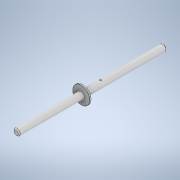
# Autodesk Inventor part: Handle
Saved by Autodesk Inventor 2022 (Build 260153000, 153)
## iProperties
Created: 2022-04-12
Part Number: Handle
Material: Generic
Document SubType Name: Modeling
Designer: Patrick
Density: 1 g/cm^3
Appearance: Default
Author: Patrick
Autodesk Inventor part; units mm, degrees
ref_plane "YZ Plane" through (0, 0, 0) normal (1, 0, 0) x (0, 1, 0)
ref_plane "XZ Plane" through (0, 0, 0) normal (0, 1, 0) x (-1, 0, 0)
ref_plane "XY Plane" through (0, 0, 0) normal (0, 0, 1) x (1, 0, 0)
sketch "Sketch1" plane through (0, 0, 0) normal (0, 1, 0) x (-1, 0, 0)
  line L0 (0, 0) -> (6, 0)
  line L1 (6, 0) -> (6, -120)
  line L2 (6, -120) -> (16, -120)
  line L3 (16, -120) -> (16, -123)
  line L4 (16, -123) -> (6, -123)
  line L5 (6, -123) -> (6, -273)
  line L6 (6, -273) -> (0, -273)
  line L7 (0, -273) -> (0, 0)
  dimension "d0" = 120
  dimension "d1" = 3
  dimension "d2" = 10
  dimension "d3" = 150
  dimension "d4" = 6
  constraints: 16 end point, 7 perpendicular, 1 coincident, 1 horizontal, 1 point on line
  measures "d0" distance of L0.end L1.end
  measures "d1" distance of L2.end L3.end
  measures "d2" distance of L4.end L3.end
  measures "d3" distance of L4.end L5.end
  measures "d4" distance of L5.end L6.end
revolve "Revolution1" add sketch "Sketch1" angle 360 about axis through (0, 0, -273) along (0, 0, 1)
sketch "Sketch3" plane through (0, 0, 0) normal (0, 1, 0) x (-1, 0, 0)
  circle A0 centre (0, -156) radius 1.5
  line L0 (-16, -123) -> (16, -123) projected
  point P0 (0, 0)
  dimension "d6" = 3
  dimension "d7" = 33
  constraints: 1 centre point
  measures "d6" diameter of A0
  measures "d7" distance from line of L0 A0.centre
extrude "Extrusion1" cut sketch "Sketch3" along normal through all both and the other way through all
chamfer "Chamfer1" distance 2 angle 45 2 edges at (6, 0, -273) (6, 0, 0)
chamfer "Chamfer2" distance 0.5 angle 45 2 edges at (16, 0, -123) (16, 0, -120)
body "Solid1"
